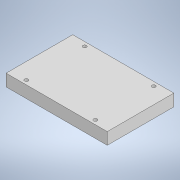
# Autodesk Inventor part: SKR PICO
Saved by Autodesk Inventor 2022 (Build 260153000, 153)
## iProperties
Created: 2022-04-23
Part Number: SKR PICO
Material: Generic
Document SubType Name: Modeling
Designer: Nick
Density: 1 g/cm^3
Appearance: Default
Author: Nick
Autodesk Inventor part; units mm, degrees
ref_plane "YZ Plane" through (0, 0, 0) normal (1, 0, 0) x (0, 1, 0)
ref_plane "XZ Plane" through (0, 0, 0) normal (0, 1, 0) x (-1, 0, 0)
ref_plane "XY Plane" through (0, 0, 0) normal (0, 0, 1) x (1, 0, 0)
sketch "Sketch1" plane through (0, 0, 0) normal (0, 1, 0) x (-1, 0, 0)
  line L0 (0, 0) -> (85, 0)
  line L1 (85, 0) -> (85, -56)
  line L2 (85, -56) -> (0, -56)
  line L3 (0, -56) -> (0, 0)
  dimension "d0" = 85
  dimension "d1" = 56
  constraints: 8 end point, 2 parallel, 1 horizontal, 1 perpendicular
  measures "d0" distance of L1.end L2.end
  measures "d1" distance of L0.end L1.end
extrude "Extrusion1" add sketch "Sketch1" along normal blind 10
sketch "Sketch2" plane through (0, 10, 0) normal (0, 1, 0) x (1, 0, 0)
  line L0 (-71.5, 52.5) -> (-13.5, 52.5) construction
  line L1 (-13.5, 52.5) -> (-13.5, 3.5) construction
  line L2 (-13.5, 3.5) -> (-71.5, 3.5) construction
  line L3 (-71.5, 3.5) -> (-71.5, 52.5) construction
  line L4 (-85, 56) -> (-85, 0) projected
  line L5 (0, 56) -> (-85, 56) projected
  point P0 (0, 0)
  point P1 (-71.5, 28)
  point P2 (-85, 28)
  point P3 (-42.5, 52.5)
  point P4 (-42.5, 56)
  dimension "d4" = 58
  dimension "d5" = 49
  constraints: 8 end point, 4 coincident, 4 midpoint, 2 parallel, 1 horizontal, 1 horizontal alignment, 1 perpendicular, 1 vertical alignment
  measures "d4" distance of L1.end L2.end
  measures "d5" distance of L0.end L1.end
hole "Hole1" at (-13.5, 10, -52.5) at (-13.5, 10, -3.5) at (-71.5, 10, -3.5) at (-71.5, 10, -52.5) direction (0, -1, 0) diameter 3 depth 10
body "Solid1"
